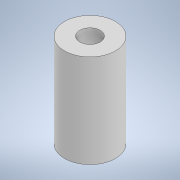
# Autodesk Inventor part: Деталь2
Saved by Autodesk Inventor 2021.2 (Build 252289000, 289)
## iProperties
Created: 2024-03-15
Part Number: Деталь2
Material: Типовые
Document SubType Name: Modeling
Designer: student
Density: 1 g/cm^3
Appearance: По умолчанию
Author: student
Autodesk Inventor part; units mm, degrees
ref_plane "YZ Plane" through (0, 0, 0) normal (1, 0, 0) x (0, 1, 0)
sketch "Эскиз1" plane through (0, 0, 0) normal (0, 1, 0) x (-1, 0, 0)
  circle A0 centre (0, 0) radius 15
  dimension "d0" = 30
  constraints: 1 centre point, 1 coincident
  measures "d0" diameter of A0
extrude "Выдавливание1" add sketch "Эскиз1" along normal blind 55
ref_plane "РабПлоскость1" through (0, 20, 0) normal (0, -1, 0) x (1, 0, 0)
sketch "Эскиз5" plane through (0, 20, 0) normal (0, -1, 0) x (1, 0, 0)
  point P0 (0, 0)
  point P1 (0, 0)
  constraints: 1 coincident
hole "Отверстие2" at (0, 20, 0) direction (0, 1, 0) diameter 20 depth 5
ref_plane "РабПлоскость2" through (0, 25, 0) normal (0, -1, 0) x (1, 0, 0)
sketch "Эскиз6" plane through (0, 25, 0) normal (0, -1, 0) x (1, 0, 0)
  point P0 (0, 0)
  point P1 (0, 0)
  constraints: 1 coincident
hole "Отверстие3" at (0, 25, 0) direction (0, 1, 0) diameter 12 end through all countersink diameter 20 countersink angle 90
sketch "Эскиз7" plane through (0, 0, 0) normal (0, -1, 0) x (1, 0, 0)
  circle A0 centre (0, 0) radius 10
  dimension "d24" = 20
  constraints: 1 centre point, 1 coincident
  measures "d24" diameter of A0
extrude "Выдавливание2" cut sketch "Эскиз7" against normal blind 20
thread "Резьба1" size "M20x1" class "6H" standard "ISO Metric profile" length 20
